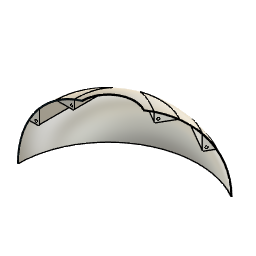
Kuppel_mit_Lasche v1 (Autodesk Fusion 360 design; units mm, degrees)
Autodesk Fusion 360 part; units mm, degrees
note: some values were not read from the file. Chosen so that the rebuilt part matches the saved one: which bodies a step acts on.
sketch "Skizze1" plane through (0, 0, 0) normal (0, 1, 0) x (1, 0, 0)
  arc A0 (-175, 0) -> (0, -175) centre (0, 0) ccw
  line L0 (0, -175) -> (0, 0)
  line L1 (0, 0) -> (-175, 0)
  constraint coincident A0.centre L0.end
  constraint vertical L0
  constraint perpendicular L0 L1
revolve "Drehen1" add sketch "Skizze1" angle 120 about axis through (0, 0, 175) along (0, 0, -1) makes body 1
shell "Schale1" thickness 1.2 removed faces 3 at (50.4782, 104.8191, 0) at (4.1508, 7.1895, 116.0729) at (-8.3017, 0, 116.0729) on bodies 1
sketch "Skizze2" plane through (0, 0, 0) normal (0, 0, 1) x (1, 0, 0)
  circle A0 centre (0, 0) radius 50
  constraint coincident A0.centre origin
extrude "Extrusion1" cut sketch "Skizze2" along normal blind 210 bodies 1
sketch "Skizze3" plane through (0, 0, 0) normal (0, -1, 0) x (1, 0, 0)
  line L0 (-50, 166.4525) -> (-50, 167.7051)
  arc A0 (-50, 167.7051) -> (-175, 0) centre (0, 0) ccw
  line L1 (-175, 0) -> (-173.8, 0)
  arc A1 (-50, 166.4525) -> (-173.8, 0) centre (0, 0) ccw
sketch "Skizze4" plane through (0, 0, 0) normal (0, 1, 0) x (1, 0, 0)
sketch "Skizze5" plane through (0, 0, 0) normal (0, 1, 0) x (1, 0, 0)
  circle A0 centre (-80, -150) radius 3.2
  line L0 (-76, -154) -> (-84, -154)
  line L1 (-84, -154) -> (-84, -146)
  line L2 (-84, -146) -> (-76, -146)
  line L3 (-76, -146) -> (-76, -154)
  circle A1 centre (-80, -150) radius 2.2
  dimension "d7" = 6.4
  dimension "d8" = 4.4
  constraint horizontal L0
  constraint vertical L1
  constraint horizontal L2
  constraint vertical L3
  constraint concentric A0 A1
  measures "d7" diameter of A0
  measures "d8" diameter of A1
sketch "Skizze7" plane through (0, 0, 0) normal (0, 1, 0) x (1, 0, 0)
  line L0 (-65, -169) -> (-115, -169)
  line L1 (-115, -169) -> (-115, -143)
  line L2 (-115, -143) -> (-65, -143)
  line L3 (-65, -143) -> (-65, -169)
  constraint horizontal L0
  constraint vertical L1
  constraint horizontal L2
  constraint vertical L3
sketch "Skizze8" plane through (0, 0, 0) normal (0, 1, 0) x (1, 0, 0)
extrude "Extrusion6" add sketch "Skizze7" along normal blind 95 separate body makes body 2
sketch "Skizze9" plane through (0, 0, 0) normal (0, -1, 0) x (1, 0, 0)
  line L0 (-115, 143) -> (-65, 143)
  line L1 (-65, 143) -> (-65, 169)
  line L2 (-65, 169) -> (-115, 169)
  line L3 (-115, 169) -> (-115, 143)
  circle A0 centre (-71, 149) radius 2.2
  dimension "d25" = 4.4
  measures "d25" diameter of A0
extrude "Extrusion7" cut sketch "Skizze9" against normal blind 8.8 contours A0 bodies 2
ref_plane "Arbeitsebene3" through (0, 0, 12.125) normal (-0.866025, 0.5, 0) x (0, 0, 1)
ref_plane "Arbeitsebene4" through (0, 0, 12.125) normal (-0.866025, -0.5, 0) x (0, 0, 1)
mirror "Spiegeln1" about plane through (0, 0, 12.125) normal (-0.866025, -0.5, 0) of bodies 2 makes body 3
sketch "Skizze10" plane through (0, 0, 0) normal (0, 1, 0) x (1, 0, 0)
sketch "Skizze11" plane through (0, 0, 0) normal (0, 1, 0) x (1, 0, 0)
sketch "Skizze12" plane through (0, 0, 0) normal (0, 1, 0) x (1, 0, 0)
  line L0 (-162.9994, -117.1237) -> (-132.9994, -117.1237)
  line L1 (-132.9994, -117.1237) -> (-132.9994, -83.1237)
  line L2 (-132.9994, -83.1237) -> (-162.9994, -83.1237)
  line L3 (-162.9994, -83.1237) -> (-162.9994, -117.1237)
  constraint horizontal L0
  constraint vertical L1
  constraint horizontal L2
  constraint vertical L3
extrude "Extrusion8" add sketch "Skizze12" along normal blind 145 separate body makes body 4
sketch "Skizze13" plane through (0, 0, 0) normal (0, -1, 0) x (1, 0, 0)
  line L0 (-162.9994, 117.1237) -> (-162.9994, 83.1237)
  line L1 (-162.9994, 83.1237) -> (-132.9994, 83.1237)
  line L2 (-132.9994, 83.1237) -> (-132.9994, 117.1237)
  line L3 (-132.9994, 117.1237) -> (-162.9994, 117.1237)
  circle A0 centre (-139, 89) radius 2.3
  dimension "d35" = 4.6
  measures "d35" diameter of A0
extrude "Extrusion9" cut sketch "Skizze13" against normal blind 12 contours A0 bodies 4
mirror "Spiegeln2" about plane through (0, 0, 12.125) normal (-0.866025, -0.5, 0) of bodies 4 makes body 5
split "Teilen1" by face at (-86.8496, 150.4279, 21.2978) of body 1 bodies 4 makes body 6 at (-162.9994, 96.6667, 94.457)
delete_body "Körper entfernen1" bodies 6
split "Teilen2" by face at (-86.8496, 150.4279, 21.2978) of body 1 bodies 2 3 5 makes body 9 at (-2.2161, 189.495, 94.457) makes body 8 at (21.7425, 100.9925, 169) makes body 7 at (-81.6667, 31.6667, 169)
delete_body "Körper entfernen2" bodies 7
delete_body "Körper entfernen3" bodies 8
delete_body "Körper entfernen4" bodies 9
fillet "Abrundung2" radius 2.5 2 edges at (-65, 38.5714, 143) (-132.9994, 38.8156, 83.1237) on bodies 2 4
chamfer "Fase1" distance 1 angle 45 1 edges at (-25, 43.3013, 167.7051) on bodies 1
fillet "Abrundung3" radius 2 2 edges at (-0.9038, 75.5773, 143) (32.8844, 134.5887, 83.1237) on bodies 3 5
extrude "Extrusion2" [suppressed]
delete_face "Fläche löschen1" [suppressed]
fillet "Abrundung1" [suppressed]
extrude "Extrusion3" [suppressed]
delete_face "Fläche löschen2" [suppressed]
extrude "Extrusion4" [suppressed]
delete_face "Fläche löschen3" [suppressed]
delete_face "Fläche löschen4" [suppressed]
sketch "Skizze6" plane through (0, 0, 0) normal (0, -1, 0) x (1, 0, 0)
  line L0 (-94.2891, 146) -> (-78.5, 146)
  arc A0 (-78.5, 146) -> (-76, 148.5) centre (-78.5, 148.5) ccw
  line L1 (-76, 148.5) -> (-76, 156.3024)
  arc A1 (-50, 166.4525) -> (-76, 156.3024) centre (0, 0) ccw
  line L2 (-50, 166.4525) -> (-50, 167.7051)
  arc A2 (-50, 167.7051) -> (-175, 0) centre (0, 0) ccw
  line L3 (-175, 0) -> (-173.8, 0)
  arc A3 (-94.2891, 146) -> (-173.8, 0) centre (0, 0) ccw
  circle A4 centre (-80.2896, 150.355) radius 2.2
  dimension "d17" = 4.4
  measures "d17" diameter of A4
extrude "Extrusion5" [suppressed]
ref_plane "Arbeitsebene2" through (0, 0, 12.125) normal (-0.866025, 0.5, 0) x (0, 0, 1)
